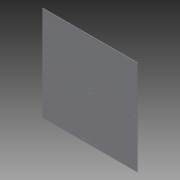
# Autodesk Inventor part: Back Funnel Piece
Saved by Autodesk Inventor 2014 (Build 180170000, 170)
## iProperties
Created: 2014-01-06
Part Number: Back Funnel Piece
Material: Aluminum 6061
Document SubType Name: Modeling
Designer: Michael
Density: 2.71 g/cm^3
Appearance: Aluminum - Flat
Author: Michael
Autodesk Inventor part; units mm, degrees
ref_plane "YZ Plane" through (0, 0, 0) normal (1, 0, 0) x (0, 1, 0)
ref_plane "XZ Plane" through (0, 0, 0) normal (0, 1, 0) x (-1, 0, 0)
ref_plane "XY Plane" through (0, 0, 0) normal (0, 0, 1) x (1, 0, 0)
sketch "Sketch1" plane through (0, 0, 0) normal (0, 0, 1) x (1, 0, 0)
  line L0 (0, 0) -> (508, 0)
  line L1 (508, 0) -> (508, 508)
  line L2 (508, 508) -> (0, 508)
  line L3 (0, 508) -> (0, 0)
  line L4 (0, 254) -> (508, 254) construction
  line L5 (254, 508) -> (254, 0) construction
  line L6 (241.3, 273.05) -> (266.7, 273.05) construction
  line L7 (266.7, 273.05) -> (266.7, 234.95) construction
  line L8 (266.7, 234.95) -> (241.3, 234.95) construction
  line L9 (241.3, 234.95) -> (241.3, 273.05) construction
  circle A0 centre (247.65, 266.7) radius 2.4892
  circle A1 centre (260.35, 266.7) radius 2.4892
  circle A2 centre (247.65, 254) radius 2.4892
  circle A3 centre (260.35, 254) radius 2.4892
  circle A4 centre (247.65, 241.3) radius 2.4892
  circle A5 centre (260.35, 241.3) radius 2.4892
  line L10 (0, 215.9) -> (19.05, 215.9) construction
  line L11 (19.05, 215.9) -> (19.05, 292.1) construction
  line L12 (19.05, 292.1) -> (0, 292.1) construction
  line L13 (0, 292.1) -> (0, 215.9) construction
  circle A6 centre (12.7, 285.75) radius 2.4892
  circle A7 centre (12.7, 222.25) radius 2.4892
  circle A8 centre (12.7, 254) radius 2.4892
  circle A9 centre (222.25, 12.7) radius 2.4892
  circle A10 centre (285.75, 12.7) radius 2.4892
  circle A11 centre (254, 12.7) radius 2.4892
  circle A12 centre (495.3, 222.25) radius 2.4892
  circle A13 centre (495.3, 285.75) radius 2.4892
  circle A14 centre (495.3, 254) radius 2.4892
  circle A15 centre (285.75, 495.3) radius 2.4892
  circle A16 centre (222.25, 495.3) radius 2.4892
  circle A17 centre (254, 495.3) radius 2.4892
  point P0 (254, 254)
  dimension "d0" = 508
  dimension "d1" = 508
  dimension "d18" = 25.4
  dimension "d19" = 38.1
  dimension "d20" = 4.9784
  dimension "d21" = 6.35
  dimension "d22" = 6.35
  dimension "d25" = 12.7
  dimension "d28" = 12.7
  dimension "d31" = 19.05
  dimension "d32" = 76.2
  dimension "d33" = 4.9784
  dimension "d34" = 6.35
  dimension "d35" = 6.35
  dimension "d36" = 6.35
  dimension "d39" = 360
  constraints: 28 end point, 18 centre point, 6 parallel, 5 midpoint, 4 horizontal, 3 perpendicular, 2 point on line, 1 equal radius, 1 symmetric about line, 1 vertical, 39 other
  measures "d0" distance of L2.end L1.end
  measures "d1" distance of L1.end L0.end
  measures "d18" distance of L7.end L8.end
  measures "d19" distance of L8.end L6.start
  measures "d20" diameter of A0
  measures "d21" distance from line of L9 A0.centre
  measures "d22" distance from line of L6 A0.centre
  measures "d25" distance of A0.centre A1.centre
  measures "d28" distance of A0.centre A2.centre
  measures "d31" distance of L10.start L10.end
  measures "d32" distance of L10.end L11.end
  measures "d33" diameter of A6
  measures "d34" distance from line of L11 A6.centre
  measures "d35" distance from line of L12 A6.centre
  measures "d36" distance from line of L11 A8.centre
extrude "Extrusion1" add sketch "Sketch1" along normal blind 1.5875
body "Solid1"
